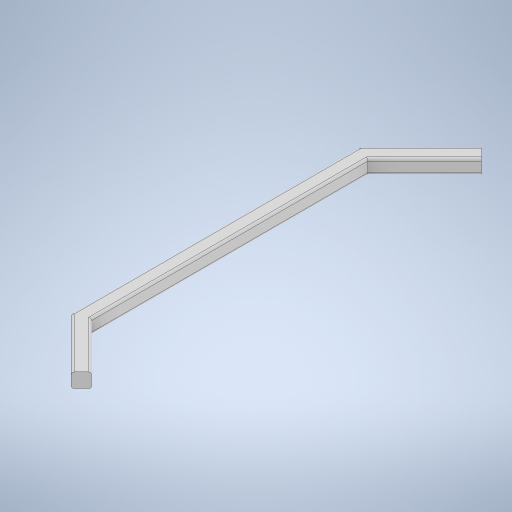
# Autodesk Inventor part: Suspension
Saved by Autodesk Inventor 2023 (Build 270158000, 158)
## iProperties
Created: 2022-11-10
Part Number: Suspension
Material: Generic
Document SubType Name: Modeling
Designer: bugme
Density: 1 g/cm^3
Appearance: Default
Author: bugme
Autodesk Inventor part; units mm, degrees
ref_plane "YZ Plane" through (0, 0, 0) normal (1, 0, 0) x (0, 1, 0)
ref_plane "XZ Plane" through (0, 0, 0) normal (0, 1, 0) x (-1, 0, 0)
ref_plane "XY Plane" through (0, 0, 0) normal (0, 0, 1) x (1, 0, 0)
sketch "Sketch1" plane through (0, 0, 0) normal (0, 1, 0) x (-1, 0, 0)
  line L0 (909.7546, -1043.3394) -> (909.7546, -1834.2484) construction
  line L1 (909.7546, -1834.2484) -> (468.795, -1834.2484) construction
  line L2 (468.795, -1834.2484) -> (468.795, -1043.3394) construction
  line L3 (468.795, -1043.3394) -> (909.7546, -1043.3394) construction
  line L4 (1047.8435, -175.8693) -> (1047.8435, -771.5628) construction
  line L5 (1047.8435, -771.5628) -> (636.4111, -771.5628) construction
  line L6 (636.4111, -771.5628) -> (636.4111, -175.8693) construction
  line L7 (636.4111, -175.8693) -> (1047.8435, -175.8693) construction
  line L8 (-89.4601, -69.3306) -> (230.5399, -69.3306) construction
  line L9 (210.5212, -775.4703) -> (125.6684, -860.3231)
  line L10 (210.5212, -775.4703) -> (330.5212, -775.4703) construction
  line L11 (125.6684, -860.3231) -> (111.5263, -846.181)
  line L12 (210.5212, -775.4703) -> (210.5212, -375.4703)
  line L13 (210.5212, -775.4703) -> (610.5212, -775.4703) construction
  line L14 (210.5212, -375.4703) -> (139.8105, -304.7596)
  line L15 (139.8105, -304.7596) -> (125.6684, -318.9018)
  line L16 (125.6684, -318.9018) -> (182.2369, -375.4703)
  line L17 (190.5212, -767.186) -> (111.5263, -846.181)
  line L18 (190.5212, -383.7546) -> (182.2369, -375.4703)
  line L19 (190.5212, -383.7546) -> (190.5212, -767.186)
  dimension "d55" = 135
  dimension "d56" = 20
  dimension "d60" = 90
  dimension "d61" = 100
  dimension "d62" = 20
  dimension "d63" = 90
  dimension "d64" = 80
  constraints: 24 end point, 3 horizontal, 2 equal length, 1 collinear, 1 perpendicular, 1 vertical, 4 other
  measures "d55" angle of L9 L10
  measures "d56" distance of L9.end L11.end
  measures "d60" angle of L13 L12
  measures "d61" distance of L12.end L14.end
  measures "d62" distance of L14.end L15.end
  measures "d63" angle of L16 L15
  measures "d64" distance of L15.end L16.end
extrude "Extrusion2" add sketch "Sketch1" along normal blind 20
fillet "Fillet1" radius 3 14 edges at (-175.1659, 20, -340.115) (-175.1659, 0, -340.115) (-210.5212, 10, -375.4703) (-210.5212, 20, -575.4703) (-210.5212, 0, -575.4703) (-190.5212, 20, -575.4703) (-153.9527, 20, -347.186) (-151.0237, 20, -806.6835) (-151.0237, 0, -806.6835) (-210.5212, 10, -775.4703) (-168.0948, 0, -817.8967) (-168.0948, 20, -817.8967) (-190.5212, 0, -575.4703) (-153.9527, 0, -347.186)
body "Solid2"
